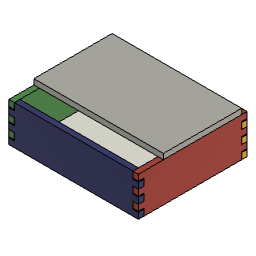
UselessBoxCardboard (Autodesk Fusion 360 design; units mm, degrees)
Autodesk Fusion 360 part; units mm, degrees
note: some values were not read from the file. Set by a fixed rule: which sketch regions a step uses.
sketch "Sketch1" plane through (0, 0, 0) normal (0, 0, 1) x (1, 0, 0) in component "bottom panel"
  line L0 (0, 0) -> (91, 0)
  line L1 (91, 0) -> (91, 75)
  line L2 (91, 75) -> (0, 75)
  line L3 (0, 75) -> (0, 0)
  dimension "d116" = 75
  dimension "d117" = 91
  constraint horizontal L0
  constraint vertical L1
  constraint horizontal L2
  constraint vertical L3
  constraint coincident L0.start L3.end
  measures "d116" distance of L0.start L2.end
  measures "d117" distance of L1.end L2.end
extrude "Extrude1" add sketch "Sketch1" against normal blind 4.2 makes body 1 in component "bottom panel"
sketch "Sketch1 (2)" plane through (0, 0, 0) normal (0, -1, 0) x (1, 0, 0) in component "front panel"
  line L0 (91, 0) -> (0, 0)
  line L1 (0, 0) -> (0, -4.2)
  line L2 (0, -4.2) -> (91, -4.2)
  line L3 (91, -4.2) -> (91, 0)
  line L4 (0, 30) -> (91, 30)
  line L5 (91, 30) -> (91, 0)
  line L6 (91, 0) -> (0, 0)
  line L7 (0, 0) -> (0, 30)
  line L8 (0, 0) -> (-4.2, 0)
  line L9 (-4.2, 0) -> (-4.2, 5.3)
  line L10 (-4.2, 5.3) -> (0, 5.3)
  line L11 (0, 5.3) -> (0, 0)
  line L12 (45.5, 30) -> (45.5, 0) construction
  line L13 (95.2, 5.3) -> (91, 5.3)
  line L14 (95.2, 0) -> (95.2, 5.3)
  line L15 (91, 0) -> (95.2, 0)
  line L16 (-4.2, 15.3) -> (0, 15.3)
  line L17 (-4.2, 10) -> (-4.2, 15.3)
  line L18 (0, 10) -> (-4.2, 10)
  line L19 (-4.2, 25.3) -> (0, 25.3)
  line L20 (-4.2, 20) -> (-4.2, 25.3)
  line L21 (0, 20) -> (-4.2, 20)
  line L22 (95.2, 15.3) -> (91, 15.3)
  line L23 (95.2, 10) -> (95.2, 15.3)
  line L24 (91, 10) -> (95.2, 10)
  line L25 (95.2, 25.3) -> (91, 25.3)
  line L26 (95.2, 20) -> (95.2, 25.3)
  line L27 (91, 20) -> (95.2, 20)
  dimension "d120" = 30
  dimension "d121" = 5.3
  dimension "d123" = 4.2
  dimension "d126" = 0
  dimension "d127" = 10
  dimension "d130" = 0
  dimension "d131" = 10
  constraint horizontal L4
  constraint vertical L5
  constraint horizontal L6
  constraint vertical L7
  constraint midpoint L0 L6
  constraint equal L0 L6
  constraint horizontal L8
  constraint vertical L9
  constraint horizontal L10
  constraint vertical L11
  constraint midpoint L4 L12.start
  constraint midpoint L6 L12.end
  constraint symmetric L0.end L12 L0.start
  constraint symmetric L8.end L12 L14.start
  constraint symmetric L9.end L12 L13.start
  constraint symmetric L10.end L12 L13.end
  measures "d120" distance of L4.end L0.start
  measures "d121" distance of L8.end L9.end
  measures "d123" distance of L9.end L10.end
extrude "Extrude1'" add sketch "Sketch1 (2)" along normal blind 4.2 separate body contours L0 L4 L5 L6 L7 L11 | L5 L13 L14 L15 | L7 L8 L9 L10 L11 | L5 L22 L23 L24 | L7 L16 L17 L18 | L5 L25 L26 L27 | L7 L19 L20 L21 makes body 2 in component "front panel"
sketch "Sketch1 (3)" plane through (0, 0, 0) normal (-1, 0, 0) x (0, -1, 0) in component "left panel"
  line L0 (0, 0) -> (-75, 0)
  line L1 (-75, 0) -> (-75, -4.2)
  line L2 (-75, -4.2) -> (0, -4.2)
  line L3 (0, -4.2) -> (0, 0)
  line L4 (0, 0) -> (-75, 0)
  line L5 (-75, 0) -> (-75, 30)
  line L6 (-75, 30) -> (0, 30)
  line L7 (0, 30) -> (0, 0)
  line L8 (0, 10) -> (4.2, 10)
  line L9 (4.2, 10) -> (4.2, 4.7)
  line L10 (4.2, 4.7) -> (0, 4.7)
  line L11 (0, 4.7) -> (0, 10)
  line L12 (-37.5, 30) -> (-37.5, 0) construction
  line L13 (-75, 10) -> (-79.2, 10)
  line L14 (-79.2, 10) -> (-79.2, 4.7)
  line L15 (-79.2, 4.7) -> (-75, 4.7)
  line L16 (4.2, 14.7) -> (0, 14.7)
  line L17 (4.2, 20) -> (4.2, 14.7)
  line L18 (0, 20) -> (4.2, 20)
  line L19 (4.2, 24.7) -> (0, 24.7)
  line L20 (4.2, 30) -> (4.2, 24.7)
  line L21 (0, 30) -> (4.2, 30)
  line L22 (-75, 20) -> (-79.2, 20)
  line L23 (-79.2, 20) -> (-79.2, 14.7)
  line L24 (-79.2, 14.7) -> (-75, 14.7)
  line L25 (-75, 30) -> (-79.2, 30)
  line L26 (-79.2, 30) -> (-79.2, 24.7)
  line L27 (-79.2, 24.7) -> (-75, 24.7)
  dimension "d134" = 75
  dimension "d135" = 30
  dimension "d136" = 4.2
  dimension "d137" = 5.3
  dimension "d138" = 4.7
  dimension "d141" = 0
  dimension "d142" = 10
  dimension "d145" = 0
  dimension "d146" = 10
  constraint horizontal L4
  constraint vertical L5
  constraint horizontal L6
  constraint vertical L7
  constraint coincident L0.start L3.end
  constraint horizontal L8
  constraint vertical L9
  constraint horizontal L10
  constraint vertical L11
  constraint coincident L7 L8.start
  constraint midpoint L6 L12.start
  constraint midpoint L4 L12.end
  constraint symmetric L8.start L12 L13.start
  constraint symmetric L8.end L12 L13.end
  constraint symmetric L9.end L12 L14.end
  constraint symmetric L10.end L12 L15.end
  measures "d134" distance of L5.end L6.end
  measures "d135" distance of L0.end L5.end
  measures "d136" distance of L8.start L8.end
  measures "d137" distance of L8.end L9.end
  measures "d138" distance of L0.start L10
extrude "Extrude1''" add sketch "Sketch1 (3)" along normal blind 4.2 separate body contours L0 L4 L5 L6 L7 L11 | L7 L8 L9 L10 L11 | L5 L13 L14 L15 | L7 L16 L17 L18 | L5 L22 L23 L24 | L7 L19 L20 L21 | L5 L25 L26 L27 makes body 3 in component "left panel"
ref_plane "WorkPlane1" through (45.5, 37.5, -2.1) normal (-1, 0, 0) x (0, 1, 0)
ref_plane "WorkPlane2" through (45.5, 37.5, -2.1) normal (0, -1, 0) x (-1, 0, 0)
mirror "MirrorComponent1" about plane through (0, 0, 0) normal (0, 0, 1) of bodies 3 makes body 4 in component "right panel"
mirror "MirrorComponent2" about plane through (0, 0, 0) normal (0, 0, 1) of bodies 2 makes body 5 in component "back panel"
sketch "Sketch1 (4)" plane through (0, 0, 30) normal (0, 0, 1) x (-1, 0, 0) in component "lid"
  line L0 (0, -75) -> (-91, -75)
  line L1 (-91, -75) -> (-91, -79.2)
  line L2 (-91, -79.2) -> (0, -79.2)
  line L3 (0, -79.2) -> (0, -75)
  line L4 (4.2, -79.2) -> (-95.2, -79.2)
  line L5 (-95.2, -79.2) -> (-95.2, -19.2)
  line L6 (-95.2, -19.2) -> (4.2, -19.2)
  line L7 (4.2, -19.2) -> (4.2, -79.2)
  dimension "d165" = 60
  dimension "d172" = 99.4
  constraint horizontal L4
  constraint vertical L5
  constraint horizontal L6
  constraint vertical L7
  constraint midpoint L2 L4
  measures "d165" distance of L4.end L5.end
  measures "d172" distance of L5.end L6.end
extrude "Extrude1'''" add sketch "Sketch1 (4)" along normal blind 4.2 separate body makes body 6 in component "lid"
component "bottom panel" placed x (1, 0, 0) y (0, 1, 0) z (0, 0, 1) at (0, 0, 0)
component "front panel" placed x (1, 0, 0) y (0, 0, 1) z (0, -1, 0) at (0, 0, 0)
component "left panel" placed x (0, 0, 1) y (0, 1, 0) z (-1, 0, 0) at (0, 0, 0)
component "right panel" placed x (0, 0, 1) y (0, 1, 0) z (-1, 0, 0) at (91, 0, 0)
component "back panel" placed x (1, 0, 0) y (0, 0, 1) z (0, -1, 0) at (0, 75, 0)
component "lid" placed x (1, 0, 0) y (0, -1, 0) z (0, 0, -1) at (0, 184.2, 30)
equation "cardboardThickness = 4.2 mm"
equation "boxFrontLen = 91 mm"
equation "boxHeight = 30 mm"
equation "boxSideLen = 75 mm"
equation "kerf = 0.3 mm"
equation "d116 = boxSideLen"
equation "d117 = boxFrontLen"
equation "d118 = -cardboardThickness"
equation "d120 = boxHeight"
equation "d121 = ( boxHeight / ( numTeeth * 2 ) ) + kerf"
equation "numTeeth = 3"
equation "d123 = cardboardThickness"
equation "d125 = numTeeth"
equation "d127 = boxHeight / ( numTeeth )"
equation "d131 = boxHeight / numTeeth"
equation "d132 = cardboardThickness"
equation "d134 = boxSideLen"
equation "d135 = boxHeight"
equation "d136 = cardboardThickness"
equation "d137 = boxHeight / ( numTeeth * 2 ) + kerf"
equation "d138 = boxHeight / ( numTeeth * 2 ) - kerf"
equation "d142 = boxHeight / numTeeth"
equation "d146 = boxHeight / numTeeth"
equation "d147 = cardboardThickness"
equation "d166 = cardboardThickness"
equation "d172 = boxFrontLen + 2 * cardboardThickness"
